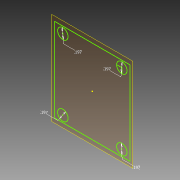
# Autodesk Inventor part: filament_feeder
Saved by Autodesk Inventor 2014 (Build 180170000, 170)
## iProperties
Created: 2014-02-16
Part Number: filament_feeder
Material: Generic
Document SubType Name: Modeling
Designer: stephen
Density: 1 g/cm^3
Appearance: Default
Author: stephen
Autodesk Inventor part; units mm, degrees
ref_plane "YZ Plane" through (0, 0, 0) normal (1, 0, 0) x (0, 1, 0)
ref_plane "XZ Plane" through (0, 0, 0) normal (0, 1, 0) x (-1, 0, 0)
ref_plane "XY Plane" through (0, 0, 0) normal (0, 0, 1) x (1, 0, 0)
ref_plane "Work Plane2" through (0, 0, 0) normal (0, 0, 1) x (1, 0, 0)
sketch "Sketch1" plane through (0, 0, 0) normal (0, 0, 1) x (1, 0, 0)
  line L0 (-0.0117, -20.0006) -> (-0.012, -20.0006)
  line L1 (-14.2652, 14.2822) -> (-14.2652, 14.1579)
  line L2 (11.2397, 17.0322) -> (11.2387, 17.0322)
  line L3 (13.9887, 16.9079) -> (13.9887, 17.0322)
  line L4 (0, 0) -> (8, 0)
  line L5 (-0.0117, -18.8998) -> (-0.0117, -18.8993)
  line L6 (-0.0117, -18.8998) -> (11.2397, -18.8993)
  line L7 (16.1373, -14.0168) -> (16.1373, 14.2822)
  line L8 (11.2275, 19.0322) -> (-11.2913, 19.0322)
  line L9 (-16.2652, 14.1579) -> (-16.2652, -14.1446)
  line L10 (-11.2913, 19.0322) -> (11.2275, 19.0322)
  line L11 (11.2397, -18.8993) -> (-11.3582, -18.8993)
  line L12 (13.9887, 14.2822) -> (11.2275, 14.27)
  line L13 (-11.2913, 14.1579) -> (-14.2652, 14.1579)
  line L14 (11.2275, 19.0322) -> (11.2275, 14.27)
  line L15 (11.2397, -14.0168) -> (11.2397, -18.8993)
  line L16 (-11.3582, -18.8993) -> (-11.3582, -14.1381)
  line L17 (-11.2913, 14.1579) -> (-11.2913, 19.0322)
  line L18 (-12.7398, -14.1446) -> (-11.3582, -14.1381)
  line L19 (11.2397, -14.0168) -> (14.1373, -14.0168)
  line L20 (18.0012, -16.7666) -> (18.0012, -16.9004)
  line L21 (17.9998, -0.0855) -> (18.0002, 0)
  line L22 (18, 16.9079) -> (18, 17.0322)
  line L23 (18.0671, 19.0322) -> (18.0671, 19.9991)
  line L24 (13.9887, 19.9331) -> (13.9887, 19.9331)
  line L25 (-0.0117, 19.9998) -> (0.1781, 19.9998)
  line L26 (-18, 20) -> (-17.9861, 20)
  line L27 (-14.2652, 20.0091) -> (-14.2559, 20.0091)
  line L28 (-18, 16.9079) -> (-18, 17.0322)
  line L29 (-17.9852, -16.7683) -> (-17.983, -16.9196)
  line L30 (-12.7398, -14.1446) -> (-16.2652, -14.1446)
  line L31 (-14.2652, 14.1579) -> (-16.2652, 14.1579)
  line L32 (13.9887, 14.2822) -> (16.1373, 14.2822)
  line L33 (14.1373, -14.0168) -> (16.1373, -14.0168)
  line L34 (-14.1063, -16.9012) -> (-13.9534, -16.9004)
  line L35 (-14.2559, -18.8993) -> (-14.2559, -18.9004)
  line L36 (-11.3582, -16.8881) -> (-11.2913, -16.8878)
  line L37 (11.2275, -16.7807) -> (11.2397, -16.7806)
  line L38 (-7.9994, -12.0931) -> (8.0006, -12.0923)
  line L39 (8.0006, -12.0923) -> (7.9994, 12.0931)
  line L40 (7.9994, 12.0931) -> (-8.0006, 12.0923)
  line L41 (-8.0006, 12.0923) -> (-7.9994, -12.0931)
  line L42 (-7.9994, -12.0931) -> (7.9994, 12.0931) construction
  line L43 (8.0006, -12.0923) -> (-8.0006, 12.0923) construction
  dimension "d11" = 8
  constraints: 88 end point, 17 parallel, 15 point on line, 10 perpendicular, 2 midpoint, 1 horizontal
  measures "d11" distance of L4.start L4.end
extrude "Extrusion1" add sketch "Sketch1" against normal blind 20 contours L41 L40 L39 L38
body "Solid1"
